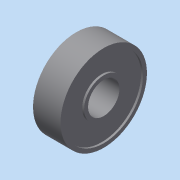
# Autodesk Inventor part: 608bearing
Saved by Autodesk Inventor 2014 SP1 (Build 180222100, 222)
## iProperties
Created: 2014-03-02
Part Number: 608bearing
Material: Generic
Document SubType Name: Modeling
Designer: Brent Yi
Density: 1 g/cm^3
Appearance: Default
d0: 0.315 in
d1: 0.866 in
d2: 0.276 in
d3: 0.00 deg
d4: 0.039 in
d5: 0.039 in
d6: 0.020 in
d7: 0.00 deg
Author: Brent Yi
Autodesk Inventor part; units mm, degrees
ref_plane "YZ Plane" through (0, 0, 0) normal (1, 0, 0) x (0, 1, 0)
ref_plane "XZ Plane" through (0, 0, 0) normal (0, 1, 0) x (-1, 0, 0)
sketch "Sketch1" plane through (0, 0, 0) normal (1, 0, 0) x (0, 1, 0)
  circle A0 centre (0, 0) radius 4
  circle A1 centre (0, 0) radius 11
  dimension "d0" = 8
  dimension "d1" = 22
  constraints: 2 centre point, 2 coincident
  measures "d0" diameter of A0
  measures "d1" diameter of A1
extrude "Extrusion1" add sketch "Sketch1" along normal blind 7
ref_plane "Work Plane1" through (3.5, 0, 0) normal (-1, 0, 0) x (0, 0, 1)
sketch "Sketch2" plane through (7, 0, 0) normal (1, 0, 0) x (0, 0, -1)
  circle A0 centre (0, 0) radius 4 projected
  circle A1 centre (0, 0) radius 11 projected
  circle A2 centre (0, 0) radius 5
  circle A3 centre (0, 0) radius 10
  dimension "d4" = 1
  dimension "d5" = 1
  constraints: 2 centre point, 2 coincident
  measures "d4" radial gap between concentric circles of A1 A3
  measures "d5" radial gap between concentric circles of A0 A2
extrude "Extrusion2" cut sketch "Sketch2" against normal blind 0.5 contours A3
mirror "Mirror1" about plane through (3.5, 0, 0) normal (-1, 0, 0) of "Extrusion2"
body "Solid1"
